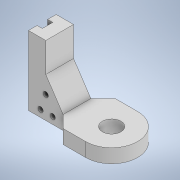
# Autodesk Inventor part: dog_bone_3
Saved by Autodesk Inventor 2020 (Build 240168000, 168)
## iProperties
Created: 2019-05-16
Part Number: dog_bone_3
Material: Generic
Document SubType Name: Modeling
Designer: psrob
Density: 1 g/cm^3
Appearance: Default
Author: psrob
Autodesk Inventor part; units mm, degrees
ref_plane "YZ Plane" through (0, 0, 0) normal (1, 0, 0) x (0, 1, 0)
ref_plane "XZ Plane" through (0, 0, 0) normal (0, 1, 0) x (-1, 0, 0)
ref_plane "XY Plane" through (0, 0, 0) normal (0, 0, 1) x (1, 0, 0)
sketch "Sketch1" plane through (0, 0, 0) normal (0, 1, 0) x (-1, 0, 0)
  circle A0 centre (0, 0) radius 15
  line L0 (0, 0) -> (0, 15)
  line L1 (0, 15) -> (40, 15)
  line L2 (40, 15) -> (40, -15)
  line L3 (40, -15) -> (0, -15)
  line L4 (0, -15) -> (0, 15)
  dimension "d0" = 30
  dimension "d1" = 15
  dimension "d2" = 40
  dimension "d3" = 30
  constraints: 10 end point, 2 parallel, 1 centre point, 1 coincident, 1 horizontal, 1 perpendicular, 1 vertical
  measures "d0" diameter of A0
  measures "d1" distance of L0.start L0.end
  measures "d2" distance of L2.end L3.end
  measures "d3" distance of L1.end L2.end
extrude "Extrusion1" add sketch "Sketch1" along normal blind 8
sketch "Sketch2" plane through (-40, 0, -15) normal (-1, 0, 0) x (0, 0, 1)
  line L0 (0, 0) -> (30, 0) projected
  line L1 (30, 0) -> (30, 8) projected
  line L2 (0, 8) -> (30, 8) projected
  line L3 (0, 0) -> (0, 8) projected
  line L4 (0, 0) -> (30, 0) projected
  line L5 (0, 0) -> (30, 0)
  line L6 (30, 0) -> (30, 40)
  line L7 (30, 40) -> (0, 40)
  line L8 (0, 40) -> (0, 0)
  point P0 (15, 0)
  dimension "d6" = 30
  dimension "d7" = 40
  constraints: 8 end point, 2 parallel, 1 horizontal, 1 perpendicular
  measures "d6" distance of L7.end L6.end
  measures "d7" distance of L6.end L5.end
extrude "Extrusion2" add sketch "Sketch2" against normal blind 5
sketch "Sketch3" plane through (-40, 40, 15) normal (0, 1, 0) x (1, 0, 0)
  line L0 (0, 0) -> (0, 30) projected
  line L1 (0, 0) -> (5, 0) projected
  line L2 (5, 30) -> (5, 0) projected
  line L3 (0, 30) -> (5, 30) projected
  line L4 (3, 18) -> (3, 12)
  line L5 (3, 12) -> (-3, 12)
  line L6 (-3, 12) -> (-3, 18)
  line L7 (-3, 18) -> (3, 18)
  line L8 (0, 30) -> (0, 0) projected
  line L9 (3, 18) -> (-3, 12) construction
  line L10 (3, 12) -> (-3, 18) construction
  point P0 (40, 15)
  point P1 (0, 15)
  dimension "d10" = 6
  dimension "d11" = 6
  constraints: 12 end point, 3 midpoint, 2 parallel, 1 perpendicular
  measures "d10" distance of L4.start L4.end
  measures "d11" distance of L4.end L5.end
extrude "Extrusion3" cut sketch "Sketch3" against normal up to surface (40 mm away) contours L5 L6 L7 L0 | L0 L7 L4 L5
sketch "Sketch4" plane through (0, 0, 0) normal (0, -1, 0) x (1, 0, 0)
  circle A0 centre (0, 0) radius 5.35
  dimension "d14" = 10.7
  constraints: 1 centre point, 1 coincident
  measures "d14" diameter of A0
extrude "Extrusion4" cut sketch "Sketch4" against normal blind 8
sketch "Sketch5" plane through (0, 0, 0) normal (0, -1, 0) x (1, 0, 0)
  circle A0 centre (0, 0) radius 5.35 projected
  line L0 (-37, -3) -> (-40, -3) projected
  line L1 (-40, -15) -> (-40, -3) projected
  line L2 (0, -15) -> (-40, -15) projected
  arc A1 (0, -15) -> (0, 15) centre (0, 0) ccw projected
  line L3 (-40, 15) -> (0, 15) projected
  line L4 (-40, 3) -> (-40, 15) projected
  line L5 (-40, 3) -> (-37, 3) projected
  line L6 (-37, 3) -> (-37, -3) projected
  line L7 (-40, -15) -> (-20, -15)
  line L8 (-20, -15) -> (-20, -8)
  line L9 (-20, -8) -> (-40, -8)
  line L10 (-40, -8) -> (-40, -15)
  line L11 (-40, 15) -> (0, 15) projected
  line L12 (-40, 15) -> (-20, 15)
  line L13 (-20, 15) -> (-20, 8)
  line L14 (-20, 8) -> (-40, 8)
  line L15 (-40, 8) -> (-40, 15)
  line L16 (-20, -8) -> (-13, -8)
  line L17 (-13, -8) -> (-13, -15)
  line L18 (-13, -15) -> (-20, -15)
  line L19 (-20, -15) -> (-20, -8)
  line L20 (-20, 8) -> (-13, 8)
  line L21 (-13, 8) -> (-13, 15)
  line L22 (-13, 15) -> (-20, 15)
  line L23 (-20, 15) -> (-20, 8)
  line L24 (-13, -15) -> (-20, -8)
  line L25 (-20, 8) -> (-13, 15)
  dimension "d17" = 20
  dimension "d18" = 7
  dimension "d19" = 20
  dimension "d20" = 7
  dimension "d21" = 7
  dimension "d22" = 7
  dimension "d23" = 7
  dimension "d24" = 7
  constraints: 36 end point, 8 parallel, 5 perpendicular, 4 horizontal
  measures "d17" distance of L9.end L8.end
  measures "d18" distance of L8.end L7.end
  measures "d19" distance of L13.end L14.end
  measures "d20" distance of L12.end L13.end
  measures "d21" distance of L17.end L18.end
  measures "d22" distance of L16.end L17.end
  measures "d23" distance of L22.end L21.end
  measures "d24" distance of L21.end L20.end
extrude "Extrusion5" cut sketch "Sketch5" against normal up to surface (40 mm away) contours L9 L8 L2 L1 | L24 L2 L8 | L4 L3 L13 L14 | L13 L3 L25
sketch "Sketch6" plane through (0, 8, 0) normal (0, 1, 0) x (1, 0, 0)
  line L0 (-20, -8) -> (-13, -15) projected
  line L1 (-13, -15) -> (0, -15) projected
  arc A0 (0, -15) -> (0, 15) centre (0, 0) ccw projected
  line L2 (0, 15) -> (-13, 15) projected
  line L3 (-13, 15) -> (-20, 8) projected
  line L4 (-20, 8) -> (-35, 8) projected
  line L5 (-35, 8) -> (-35, -8) projected
  line L6 (-35, -8) -> (-20, -8) projected
  circle A1 centre (0, 0) radius 5.35 projected
  line L7 (-35, 8) -> (-35, -8) projected
  line L8 (-35, -8) -> (-30, -8)
  line L9 (-30, -8) -> (-30, 8)
  line L10 (-30, 8) -> (-35, 8)
  line L11 (-35, 8) -> (-35, -8)
  dimension "d27" = 5
  dimension "d28" = 16
  constraints: 8 end point, 2 parallel, 1 horizontal, 1 perpendicular
  measures "d27" distance of L10.end L9.end
  measures "d28" distance of L9.end L8.end
extrude "Extrusion6" add sketch "Sketch6" along normal up to surface (32 mm away) contours L6 L5 L4 L9
sketch "Sketch8" plane through (-40, 0, 8) normal (0, 0, 1) x (1, 0, 0)
  line L0 (10, 8) -> (10, 40) projected
  line L1 (0, 40) -> (10, 40) projected
  line L2 (0, 0) -> (0, 40) projected
  line L3 (20, 0) -> (0, 0) projected
  line L4 (20, 0) -> (20, 8) projected
  line L5 (10, 8) -> (20, 8) projected
  line L6 (10, 8) -> (10, 40) projected
  line L7 (10, 8) -> (10, 23)
  line L8 (10, 23) -> (20, 8)
  point P0 (40, 0)
  dimension "d34" = 15
  constraints: 4 end point, 1 point on line
  measures "d34" distance of L0.start L7.end
extrude "Extrusion8" add sketch "Sketch8" against normal up to surface (16 mm away) contours L0 L8 L5
sketch "Sketch9" plane through (-20, 0, -8) normal (0, 0, -1) x (-1, 0, 0)
  line L0 (0, 0) -> (0, 8) projected
  line L1 (20, 0) -> (0, 0) projected
  line L2 (20, 40) -> (20, 0) projected
  line L3 (10, 40) -> (20, 40) projected
  line L4 (10, 23) -> (10, 40) projected
  line L5 (10, 23) -> (0, 8) projected
  line L6 (20, 0) -> (0, 0) projected
  line L7 (0, 0) -> (0, 4)
  line L8 (0, 0) -> (0, 8) projected
  line L9 (0, 4) -> (6, 4)
  line L10 (6, 4) -> (13, 4)
  circle A0 centre (6, 4) radius 1.5
  circle A1 centre (13, 4) radius 1.5
  line L11 (13, 4) -> (13, 13)
  line L12 (13, 13) -> (10, 13)
  circle A2 centre (10, 13) radius 1.5
  point P0 (-20, 0)
  dimension "d37" = 4
  dimension "d38" = 6
  dimension "d39" = 7
  dimension "d40" = 3
  dimension "d41" = 3
  dimension "d42" = 9
  dimension "d43" = 3
  dimension "d44" = 3
  constraints: 10 end point, 3 centre point, 3 coincident, 2 perpendicular, 1 midpoint, 1 point on line, 1 vertical
  measures "d37" distance of L0.start L7.end
  measures "d38" distance of L7.end L9.end
  measures "d39" distance of L9.end L10.end
  measures "d40" diameter of A0
  measures "d41" diameter of A1
  measures "d42" distance of L11.start L11.end
  measures "d43" distance of L11.end L12.end
  measures "d44" diameter of A2
extrude "Extrusion9" cut sketch "Sketch9" against normal up to surface (16 mm away) contours A0 L10 L9 | L9 L10 A0 | A1 L11 L10 | L10 L11 A1 | A2
body "Solid1"
